Autodesk Fusion 360 part; units mm, degrees
(part 2 of 4)
sketch "Esboço21" plane through (0, 0, 25.51) normal (0, 0, 1) x (-1, 0, 0)
  arc A0 (-264.8266, 72.716) -> (-256.8894, 72.716) centre (-260.858, 77.216) ccw
  line L0 (-264.8266, 72.716) -> (-256.8894, 72.716)
  arc A1 (-203.4723, 131.348) -> (-203.0106, 132.848) centre (-208.9267, 133.848) ccw
  line L1 (-203.4723, 131.348) -> (-214.381, 131.348)
  arc A2 (-214.8427, 132.848) -> (-214.381, 131.348) centre (-208.9267, 133.848) ccw
  line L2 (-214.8427, 132.848) -> (-203.0106, 132.848)
  arc A3 (-212.8953, 129.348) -> (-204.958, 129.348) centre (-208.9267, 133.848) ccw
  line L3 (-212.8953, 129.348) -> (-204.958, 129.348)
  line L4 (-255.4036, 74.716) -> (-266.3124, 74.716)
  arc A4 (-266.7741, 76.216) -> (-266.3124, 74.716) centre (-260.858, 77.216) ccw
  line L5 (-266.7741, 76.216) -> (-254.9419, 76.216)
  arc A5 (-255.4036, 74.716) -> (-254.9419, 76.216) centre (-260.858, 77.216) ccw
  line L6 (-203.0106, 134.848) -> (-214.8427, 134.848)
  arc A6 (-214.381, 136.348) -> (-214.8427, 134.848) centre (-208.9267, 133.848) ccw
  line L7 (-214.381, 136.348) -> (-203.4723, 136.348)
  arc A7 (-203.0106, 134.848) -> (-203.4723, 136.348) centre (-208.9267, 133.848) ccw
  line L8 (-254.9419, 78.216) -> (-266.7741, 78.216)
  arc A8 (-266.3124, 79.716) -> (-266.7741, 78.216) centre (-260.858, 77.216) ccw
  line L9 (-266.3124, 79.716) -> (-255.4036, 79.716)
  arc A9 (-254.9419, 78.216) -> (-255.4036, 79.716) centre (-260.858, 77.216) ccw
  circle A10 centre (-239.522, 60.452) radius 2.5
  circle A11 centre (-207.899, 118.364) radius 2.5
  line L10 (-257.756, 60.626) -> (-257.806, 60.626)
  line L11 (-257.806, 60.626) -> (-257.806, 60.226)
  line L12 (-257.806, 60.226) -> (-265.506, 60.226)
  line L13 (-265.506, 60.226) -> (-265.506, 60.626)
  line L14 (-265.506, 60.626) -> (-265.556, 60.626)
  line L15 (-265.556, 60.626) -> (-265.556, 63.326)
  line L16 (-265.556, 63.326) -> (-265.506, 63.326)
  line L17 (-265.506, 63.326) -> (-265.506, 63.726)
  line L18 (-265.506, 63.726) -> (-257.806, 63.726)
  line L19 (-257.806, 63.726) -> (-257.806, 63.326)
  line L20 (-257.806, 63.326) -> (-257.756, 63.326)
  line L21 (-257.756, 63.326) -> (-257.756, 60.626)
  line L22 (-204.958, 138.348) -> (-212.8953, 138.348)
  arc A12 (-204.958, 138.348) -> (-212.8953, 138.348) centre (-208.9267, 133.848) ccw
  line L23 (-256.8894, 81.716) -> (-264.8266, 81.716)
  arc A13 (-256.8894, 81.716) -> (-264.8266, 81.716) centre (-260.858, 77.216) ccw
  line L24 (-271.5, 38) -> (-166.5, 38)
  line L25 (-166.5, 38) -> (-166.5, 143)
  line L26 (-166.5, 143) -> (-271.5, 143)
  line L27 (-271.5, 143) -> (-271.5, 38)
  spline S0 degree 3 poles (-184.8623, 130.1732) (-186.1405, 129.7688) (-187.3103, 128.5701) (-188.1551, 126.8082) knots 0 0 0 0 1 1 1 1
  spline S1 degree 3 poles (-188.1551, 126.8082) (-188.805, 125.4434) (-189.6138, 123.1543) (-190.1698, 121.118) knots 0 0 0 0 1 1 1 1
  spline S2 degree 3 poles (-190.1698, 121.118) (-190.6175, 119.4716) (-191.5201, 114.6263) (-191.614, 113.3771) knots 0 0 0 0 1 1 1 1
  spline S3 degree 3 poles (-191.614, 113.3771) (-191.7079, 112.1206) (-191.6429, 109.7088) (-191.4985, 109.0589) knots 0 0 0 0 1 1 1 1
  line L28 (-191.4985, 109.0589) -> (-191.3901, 108.6112)
  line L29 (-191.3901, 108.6112) -> (-191.7006, 108.1851)
  spline S4 degree 3 poles (-191.7006, 108.1851) (-191.8667, 107.9541) (-192.0689, 107.6363) (-192.1556, 107.4919) knots 0 0 0 0 1 1 1 1
  line L30 (-192.1556, 107.4919) -> (-192.3072, 107.2175)
  line L31 (-192.3072, 107.2175) -> (-192.6105, 107.788)
  spline S5 degree 3 poles (-192.6105, 107.788) (-193.4842, 109.4127) (-195.0368, 110.8497) (-196.5315, 111.4274) knots 0 0 0 0 1 1 1 1
  spline S6 degree 3 poles (-196.5315, 111.4274) (-197.1742, 111.6729) (-198.1418, 111.8606) (-198.8061, 111.8606) knots 0 0 0 0 1 1 1 1
  spline S7 degree 3 poles (-198.8061, 111.8606) (-199.2611, 111.8606) (-199.2827, 111.8679) (-199.651, 112.2) knots 0 0 0 0 1 1 1 1
  spline S8 degree 3 poles (-199.651, 112.2) (-200.4742, 112.951) (-201.7379, 113.6298) (-202.8355, 113.9186) knots 0 0 0 0 1 1 1 1
  spline S9 degree 3 poles (-202.8355, 113.9186) (-203.0738, 113.9836) (-203.6226, 114.0703) (-204.0631, 114.1136) knots 0 0 0 0 1 1 1 1
  spline S10 degree 3 poles (-204.0631, 114.1136) (-206.5038, 114.3663) (-208.93, 113.3915) (-210.2876, 111.6079) knots 0 0 0 0 1 1 1 1
  spline S11 degree 3 poles (-210.2876, 111.6079) (-211.0386, 110.6258) (-211.5946, 109.2322) (-211.7535, 107.9324) knots 0 0 0 0 1 1 1 1
  spline S12 degree 3 poles (-211.7535, 107.9324) (-211.8762, 106.972) (-211.804, 105.3112) (-211.609, 104.5024) knots 0 0 0 0 1 1 1 1
  spline S13 degree 3 poles (-211.609, 104.5024) (-211.5296, 104.163) (-211.4863, 103.867) (-211.5152, 103.8381) knots 0 0 0 0 1 1 1 1
  spline S14 degree 3 poles (-211.5152, 103.8381) (-211.5513, 103.8164) (-211.8329, 103.737) (-212.1506, 103.6648) knots 0 0 0 0 1 1 1 1
  spline S15 degree 3 poles (-212.1506, 103.6648) (-212.8366, 103.5203) (-214.6491, 102.9282) (-215.5084, 102.5672) knots 0 0 0 0 1 1 1 1
  spline S16 degree 3 poles (-215.5084, 102.5672) (-216.4255, 102.1772) (-216.5627, 102.1989) (-217.8191, 102.8416) knots 0 0 0 0 1 1 1 1
  spline S17 degree 3 poles (-217.8191, 102.8416) (-218.3968, 103.1376) (-219.0467, 103.4265) (-219.2633, 103.477) knots 0 0 0 0 1 1 1 1
  spline S18 degree 3 poles (-219.2633, 103.477) (-219.5089, 103.5348) (-220.2598, 103.5853) (-221.2419, 103.5998) knots 0 0 0 0 1 1 1 1
  line L32 (-221.2419, 103.5998) -> (-222.8161, 103.6214)
  line L33 (-222.8161, 103.6214) -> (-223.3721, 103.9031)
  spline S19 degree 3 poles (-223.3721, 103.9031) (-224.1231, 104.2858) (-224.8163, 104.5024) (-225.459, 104.5602) knots 0 0 0 0 1 1 1 1
  line L34 (-225.459, 104.5602) -> (-226.0006, 104.6035)
  line L35 (-226.0006, 104.6035) -> (-226.4699, 105.6867)
  spline S20 degree 3 poles (-226.4699, 105.6867) (-226.7227, 106.286) (-227.3003, 107.5641) (-227.7481, 108.539) knots 0 0 0 0 1 1 1 1
  spline S21 degree 3 poles (-227.7481, 108.539) (-228.1958, 109.5138) (-228.9756, 111.2035) (-229.4739, 112.2939) knots 0 0 0 0 1 1 1 1
  spline S22 degree 3 poles (-229.4739, 112.2939) (-229.9794, 113.3843) (-230.6148, 114.7346) (-230.8892, 115.2906) knots 0 0 0 0 1 1 1 1
  spline S23 degree 3 poles (-230.8892, 115.2906) (-232.3695, 118.2874) (-234.0304, 120.6414) (-236.1028, 122.6633) knots 0 0 0 0 1 1 1 1
  spline S24 degree 3 poles (-236.1028, 122.6633) (-237.8214, 124.3458) (-239.0345, 125.1546) (-240.9842, 125.92) knots 0 0 0 0 1 1 1 1
  spline S25 degree 3 poles (-240.9842, 125.92) (-242.1901, 126.3894) (-242.7678, 126.5193) (-243.6704, 126.5193) knots 0 0 0 0 1 1 1 1
  spline S26 degree 3 poles (-243.6704, 126.5193) (-246.3061, 126.5193) (-248.2197, 124.909) (-248.2197, 122.685) knots 0 0 0 0 1 1 1 1
  spline S27 degree 3 poles (-248.2197, 122.685) (-248.2197, 121.9268) (-248.1114, 121.4646) (-247.7864, 120.7786) knots 0 0 0 0 1 1 1 1
  spline S28 degree 3 poles (-247.7864, 120.7786) (-247.2737, 119.7316) (-246.8044, 119.3272) (-244.9341, 118.3523) knots 0 0 0 0 1 1 1 1
  spline S29 degree 3 poles (-244.9341, 118.3523) (-243.6777, 117.7025) (-243.4755, 117.5725) (-242.8256, 117.0453) knots 0 0 0 0 1 1 1 1
  spline S30 degree 3 poles (-242.8256, 117.0453) (-241.2875, 115.7961) (-239.6411, 113.7959) (-238.4063, 111.6873) knots 0 0 0 0 1 1 1 1
  spline S31 degree 3 poles (-238.4063, 111.6873) (-237.973, 110.9436) (-237.0704, 109.16) (-236.6516, 108.214) knots 0 0 0 0 1 1 1 1
  spline S32 degree 3 poles (-236.6516, 108.214) (-236.2833, 107.3836) (-235.1496, 104.5674) (-235.1496, 104.488) knots 0 0 0 0 1 1 1 1
  spline S33 degree 3 poles (-235.1496, 104.488) (-235.1496, 104.4519) (-235.4457, 104.423) (-235.7995, 104.423) knots 0 0 0 0 1 1 1 1
  spline S34 degree 3 poles (-235.7995, 104.423) (-236.1606, 104.423) (-236.7021, 104.3724) (-236.9982, 104.3074) knots 0 0 0 0 1 1 1 1
  spline S35 degree 3 poles (-236.9982, 104.3074) (-237.5037, 104.2063) (-237.5614, 104.2063) (-237.7275, 104.3147) knots 0 0 0 0 1 1 1 1
  spline S36 degree 3 poles (-237.7275, 104.3147) (-238.5074, 104.8273) (-240.096, 104.9068) (-241.0781, 104.488) knots 0 0 0 0 1 1 1 1
  line L36 (-241.0781, 104.488) -> (-241.4319, 104.3363)
  line L37 (-241.4319, 104.3363) -> (-242.3129, 104.9068)
  spline S37 degree 3 poles (-242.3129, 104.9068) (-243.5332, 105.6939) (-243.7787, 105.8311) (-244.4359, 106.0549) knots 0 0 0 0 1 1 1 1
  spline S38 degree 3 poles (-244.4359, 106.0549) (-244.9197, 106.2282) (-245.1219, 106.2571) (-245.7645, 106.2571) knots 0 0 0 0 1 1 1 1
  spline S39 degree 3 poles (-245.7645, 106.2571) (-246.6383, 106.2499) (-247.1654, 106.0983) (-247.8803, 105.6217) knots 0 0 0 0 1 1 1 1
  spline S40 degree 3 poles (-247.8803, 105.6217) (-249.5122, 104.5385) (-249.7505, 102.1844) (-248.3858, 100.668) knots 0 0 0 0 1 1 1 1
  spline S41 degree 3 poles (-248.3858, 100.668) (-248.1908, 100.4442) (-247.6276, 100.0181) (-247.0354, 99.621) knots 0 0 0 0 1 1 1 1
  spline S42 degree 3 poles (-247.0354, 99.621) (-246.0534, 98.9783) (-245.2518, 98.4728) (-238.724, 94.3857) knots 0 0 0 0 1 1 1 1
  spline S43 degree 3 poles (-238.724, 94.3857) (-232.7811, 90.6669) (-227.6758, 87.4391) (-227.5459, 87.3091) knots 0 0 0 0 1 1 1 1
  spline S44 degree 3 poles (-227.5459, 87.3091) (-227.5098, 87.2802) (-227.7481, 86.977) (-228.0658, 86.6376) knots 0 0 0 0 1 1 1 1
  spline S45 degree 3 poles (-228.0658, 86.6376) (-228.759, 85.8866) (-229.3583, 85.15) (-229.8783, 84.4207) knots 0 0 0 0 1 1 1 1
  spline S46 degree 3 poles (-229.8783, 84.4207) (-230.0877, 84.1246) (-230.3043, 83.843) (-230.3621, 83.7997) knots 0 0 0 0 1 1 1 1
  spline S47 degree 3 poles (-230.3621, 83.7997) (-230.4776, 83.6986) (-230.687, 83.7491) (-231.4308, 84.0163) knots 0 0 0 0 1 1 1 1
  spline S48 degree 3 poles (-231.4308, 84.0163) (-231.8785, 84.1824) (-232.0518, 84.2041) (-232.8822, 84.2041) knots 0 0 0 0 1 1 1 1
  spline S49 degree 3 poles (-232.8822, 84.2041) (-233.8859, 84.2041) (-234.3336, 84.1102) (-235.0774, 83.7347) knots 0 0 0 0 1 1 1 1
  spline S50 degree 3 poles (-235.0774, 83.7347) (-235.2579, 83.6481) (-235.6767, 83.482) (-236.0161, 83.3737) knots 0 0 0 0 1 1 1 1
  spline S51 degree 3 poles (-236.0161, 83.3737) (-236.3555, 83.2653) (-236.8177, 83.0776) (-237.0487, 82.9548) knots 0 0 0 0 1 1 1 1
  spline S52 degree 3 poles (-237.0487, 82.9548) (-237.807, 82.5577) (-238.5291, 81.6984) (-238.7601, 80.9113) knots 0 0 0 0 1 1 1 1
  spline S53 degree 3 poles (-238.7601, 80.9113) (-238.8396, 80.6513) (-238.8901, 80.6008) (-239.1284, 80.5286) knots 0 0 0 0 1 1 1 1
  spline S54 degree 3 poles (-239.1284, 80.5286) (-239.28, 80.4852) (-239.5833, 80.348) (-239.8072, 80.2325) knots 0 0 0 0 1 1 1 1
  spline S55 degree 3 poles (-239.8072, 80.2325) (-240.5148, 79.8642) (-239.8722, 79.5321) (-245.8728, 83.3231) knots 0 0 0 0 1 1 1 1
  spline S56 degree 3 poles (-245.8728, 83.3231) (-248.5446, 85.0128) (-248.6096, 85.0489) (-248.9851, 85.1861) knots 0 0 0 0 1 1 1 1
  spline S57 degree 3 poles (-248.9851, 85.1861) (-249.5195, 85.3811) (-250.6532, 85.3594) (-251.202, 85.15) knots 0 0 0 0 1 1 1 1
  spline S58 degree 3 poles (-251.202, 85.15) (-252.1985, 84.7601) (-252.9856, 83.9947) (-253.3177, 83.0776) knots 0 0 0 0 1 1 1 1
  spline S59 degree 3 poles (-253.3177, 83.0776) (-253.491, 82.6082) (-253.5055, 82.471) (-253.4766, 81.7995) knots 0 0 0 0 1 1 1 1
  spline S60 degree 3 poles (-253.4766, 81.7995) (-253.4549, 81.1063) (-253.4333, 81.0052) (-253.1805, 80.5069) knots 0 0 0 0 1 1 1 1
  spline S61 degree 3 poles (-253.1805, 80.5069) (-252.5379, 79.1927) (-251.3969, 78.2467) (-248.4002, 76.5137) knots 0 0 0 0 1 1 1 1
  spline S62 degree 3 poles (-248.4002, 76.5137) (-247.7214, 76.1237) (-246.5372, 75.3944) (-245.7645, 74.8889) knots 0 0 0 0 1 1 1 1
  spline S63 degree 3 poles (-245.7645, 74.8889) (-244.9919, 74.3835) (-243.8871, 73.6902) (-243.3094, 73.3364) knots 0 0 0 0 1 1 1 1
  spline S64 degree 3 poles (-243.3094, 73.3364) (-242.7317, 72.9898) (-240.7676, 71.7911) (-238.9407, 70.6791) knots 0 0 0 0 1 1 1 1
  spline S65 degree 3 poles (-238.9407, 70.6791) (-237.1137, 69.567) (-234.998, 68.2817) (-234.247, 67.8195) knots 0 0 0 0 1 1 1 1
  spline S66 degree 3 poles (-234.247, 67.8195) (-233.4888, 67.3646) (-231.9074, 66.3753) (-230.7231, 65.6316) knots 0 0 0 0 1 1 1 1
  spline S67 degree 3 poles (-230.7231, 65.6316) (-228.2752, 64.0791) (-227.8564, 63.8552) (-226.9537, 63.5808) knots 0 0 0 0 1 1 1 1
  spline S68 degree 3 poles (-226.9537, 63.5808) (-226.3761, 63.4075) (-226.1522, 63.3858) (-224.9752, 63.3497) knots 0 0 0 0 1 1 1 1
  spline S69 degree 3 poles (-224.9752, 63.3497) (-223.5671, 63.3136) (-222.9027, 63.3858) (-222.1373, 63.6313) knots 0 0 0 0 1 1 1 1
  line L38 (-222.1373, 63.6313) -> (-221.704, 63.7758)
  line L39 (-221.704, 63.7758) -> (-221.408, 63.5014)
  spline S70 degree 3 poles (-221.408, 63.5014) (-221.2419, 63.3497) (-220.7436, 63.0031) (-220.3104, 62.7359) knots 0 0 0 0 1 1 1 1
  spline S71 degree 3 poles (-220.3104, 62.7359) (-219.8699, 62.4615) (-219.09, 61.9777) (-218.5773, 61.6528) knots 0 0 0 0 1 1 1 1
  spline S72 degree 3 poles (-218.5773, 61.6528) (-218.0574, 61.3278) (-216.8443, 60.5552) (-215.8695, 59.9486) knots 0 0 0 0 1 1 1 1
  spline S73 degree 3 poles (-215.8695, 59.9486) (-214.8946, 59.3348) (-213.3204, 58.3383) (-212.3672, 57.739) knots 0 0 0 0 1 1 1 1
  spline S74 degree 3 poles (-212.3672, 57.739) (-210.3454, 56.4536) (-209.7099, 56.1142) (-208.8073, 55.8543) knots 0 0 0 0 1 1 1 1
  spline S75 degree 3 poles (-208.8073, 55.8543) (-208.1718, 55.6738) (-208.0852, 55.6665) (-206.8215, 55.7027) knots 0 0 0 0 1 1 1 1
  spline S76 degree 3 poles (-206.8215, 55.7027) (-205.4206, 55.7315) (-205.1751, 55.7893) (-204.2436, 56.2587) knots 0 0 0 0 1 1 1 1
  spline S77 degree 3 poles (-204.2436, 56.2587) (-203.2543, 56.7569) (-202.1206, 57.7101) (-201.4346, 58.6127) knots 0 0 0 0 1 1 1 1
  spline S78 degree 3 poles (-201.4346, 58.6127) (-201.2469, 58.8582) (-200.9002, 59.2193) (-200.6692, 59.4215) knots 0 0 0 0 1 1 1 1
  spline S79 degree 3 poles (-200.6692, 59.4215) (-199.3116, 60.5624) (-197.9829, 62.2305) (-197.0442, 63.978) knots 0 0 0 0 1 1 1 1
  spline S80 degree 3 poles (-197.0442, 63.978) (-196.8637, 64.3173) (-196.6976, 64.6134) (-196.6904, 64.6278) knots 0 0 0 0 1 1 1 1
  spline S81 degree 3 poles (-196.6904, 64.6278) (-196.6759, 64.6423) (-196.2355, 64.3751) (-195.7083, 64.0429) knots 0 0 0 0 1 1 1 1
  spline S82 degree 3 poles (-195.7083, 64.0429) (-193.4193, 62.5771) (-192.3578, 61.9344) (-191.7656, 61.6528) knots 0 0 0 0 1 1 1 1
  line L40 (-191.7656, 61.6528) -> (-191.1374, 61.3495)
  line L41 (-191.1374, 61.3495) -> (-190.047, 61.3278)
  spline S83 degree 3 poles (-190.047, 61.3278) (-189.0361, 61.3062) (-188.9133, 61.3134) (-188.3645, 61.4867) knots 0 0 0 0 1 1 1 1
  spline S84 degree 3 poles (-188.3645, 61.4867) (-188.0396, 61.5878) (-187.6496, 61.6744) (-187.498, 61.6744) knots 0 0 0 0 1 1 1 1
  spline S85 degree 3 poles (-187.498, 61.6744) (-186.5737, 61.6744) (-185.245, 62.5626) (-184.6024, 63.6097) knots 0 0 0 0 1 1 1 1
  line L42 (-184.6024, 63.6097) -> (-184.3857, 63.9707)
  line L43 (-184.3857, 63.9707) -> (-182.5227, 64.0068)
  spline S86 degree 3 poles (-182.5227, 64.0068) (-178.3273, 64.1007) (-178.0962, 64.1296) (-177.0853, 64.6351) knots 0 0 0 0 1 1 1 1
  spline S87 degree 3 poles (-177.0853, 64.6351) (-176.5148, 64.9311) (-175.8433, 65.5882) (-175.6122, 66.1009) knots 0 0 0 0 1 1 1 1
  spline S88 degree 3 poles (-175.6122, 66.1009) (-175.3739, 66.6136) (-175.2584, 67.509) (-175.3089, 68.455) knots 0 0 0 0 1 1 1 1
  spline S89 degree 3 poles (-175.3089, 68.455) (-175.3739, 69.8703) (-175.836, 71.0907) (-176.6809, 72.08) knots 0 0 0 0 1 1 1 1
  spline S90 degree 3 poles (-176.6809, 72.08) (-176.9409, 72.376) (-177.1719, 72.701) (-177.208, 72.8021) knots 0 0 0 0 1 1 1 1
  spline S91 degree 3 poles (-177.208, 72.8021) (-177.3525, 73.2425) (-177.2153, 81.2146) (-177.0131, 83.6986) knots 0 0 0 0 1 1 1 1
  spline S92 degree 3 poles (-177.0131, 83.6986) (-176.8542, 85.6916) (-177.1791, 87.0203) (-178.0168, 87.7496) knots 0 0 0 0 1 1 1 1
  spline S93 degree 3 poles (-178.0168, 87.7496) (-178.3562, 88.0529) (-178.9411, 88.3128) (-179.3888, 88.3706) knots 0 0 0 0 1 1 1 1
  line L44 (-179.3888, 88.3706) -> (-179.7426, 88.4067)
  line L45 (-179.7426, 88.4067) -> (-179.7859, 89.1144)
  spline S94 degree 3 poles (-179.7859, 89.1144) (-179.8437, 90.0964) (-180.0892, 90.7969) (-180.5441, 91.2951) knots 0 0 0 0 1 1 1 1
  line L46 (-180.5441, 91.2951) -> (-180.7247, 91.4973)
  line L47 (-180.7247, 91.4973) -> (-180.4647, 92.27)
  spline S95 degree 3 poles (-180.4647, 92.27) (-179.9954, 93.6636) (-179.8365, 94.9562) (-179.9737, 96.1838) knots 0 0 0 0 1 1 1 1
  spline S96 degree 3 poles (-179.9737, 96.1838) (-180.2264, 98.3501) (-181.1652, 99.982) (-182.7538, 101.0219) knots 0 0 0 0 1 1 1 1
  spline S97 degree 3 poles (-182.7538, 101.0219) (-183.4181, 101.4551) (-184.3569, 101.8595) (-184.9634, 101.9678) knots 0 0 0 0 1 1 1 1
  spline S98 degree 3 poles (-184.9634, 101.9678) (-185.7361, 102.1122) (-185.7216, 102.0978) (-185.4617, 102.4733) knots 0 0 0 0 1 1 1 1
  spline S99 degree 3 poles (-185.4617, 102.4733) (-185.1078, 103.0004) (-184.7757, 103.7009) (-184.6096, 104.2785) knots 0 0 0 0 1 1 1 1
  spline S100 degree 3 poles (-184.6096, 104.2785) (-184.4002, 105.0151) (-184.3424, 106.1127) (-184.4796, 106.7698) knots 0 0 0 0 1 1 1 1
  line L48 (-184.4796, 106.7698) -> (-184.5879, 107.2753)
  line L49 (-184.5879, 107.2753) -> (-184.2774, 107.6724)
  spline S101 degree 3 poles (-184.2774, 107.6724) (-183.2448, 109.0228) (-182.7754, 110.3153) (-181.4901, 115.3917) knots 0 0 0 0 1 1 1 1
  spline S102 degree 3 poles (-181.4901, 115.3917) (-181.1724, 116.6482) (-180.7824, 118.1646) (-180.6308, 118.7712) knots 0 0 0 0 1 1 1 1
  spline S103 degree 3 poles (-180.6308, 118.7712) (-179.9304, 121.4935) (-179.656, 123.3565) (-179.7065, 125.1112) knots 0 0 0 0 1 1 1 1
  spline S104 degree 3 poles (-179.7065, 125.1112) (-179.7498, 126.4905) (-179.8726, 127.1115) (-180.2914, 127.9563) knots 0 0 0 0 1 1 1 1
  spline S105 degree 3 poles (-180.2914, 127.9563) (-180.7969, 129.0034) (-181.5912, 129.7038) (-182.7032, 130.0937) knots 0 0 0 0 1 1 1 1
  spline S106 degree 3 poles (-182.7032, 130.0937) (-183.0932, 130.2382) (-183.3315, 130.2671) (-183.8803, 130.2671) knots 0 0 0 0 1 1 1 1
  spline S107 degree 3 poles (-183.8803, 130.2671) (-184.2558, 130.2671) (-184.6962, 130.2237) (-184.8623, 130.1732) knots 0 0 0 0 1 1 1 1
  spline S108 degree 3 poles (-182.9993, 129.1117) (-181.9523, 128.7651) (-181.2301, 127.9347) (-180.8835, 126.6926) knots 0 0 0 0 1 1 1 1
  spline S109 degree 3 poles (-180.8835, 126.6926) (-180.7247, 126.115) (-180.6597, 124.3025) (-180.768, 123.3349) knots 0 0 0 0 1 1 1 1
  spline S110 degree 3 poles (-180.768, 123.3349) (-180.9124, 122.0567) (-181.2013, 120.6125) (-181.6056, 119.0456) knots 0 0 0 0 1 1 1 1
  spline S111 degree 3 poles (-181.6056, 119.0456) (-181.714, 118.6484) (-182.0822, 117.1898) (-182.4361, 115.7961) knots 0 0 0 0 1 1 1 1
  spline S112 degree 3 poles (-182.4361, 115.7961) (-183.1582, 112.951) (-183.7792, 110.7919) (-184.0969, 110.0265) knots 0 0 0 0 1 1 1 1
  spline S113 degree 3 poles (-184.0969, 110.0265) (-184.393, 109.3261) (-184.8768, 108.5173) (-185.3173, 107.9974) knots 0 0 0 0 1 1 1 1
  spline S114 degree 3 poles (-185.3173, 107.9974) (-185.7216, 107.528) (-185.7289, 107.4991) (-185.5844, 107.0153) knots 0 0 0 0 1 1 1 1
  spline S115 degree 3 poles (-185.5844, 107.0153) (-185.1945, 105.73) (-185.5267, 104.0619) (-186.4149, 102.8849) knots 0 0 0 0 1 1 1 1
  spline S116 degree 3 poles (-186.4149, 102.8849) (-187.6352, 101.2602) (-189.5488, 101.0002) (-190.8269, 102.2783) knots 0 0 0 0 1 1 1 1
  spline S117 degree 3 poles (-190.8269, 102.2783) (-191.4768, 102.9282) (-191.9028, 104.1486) (-191.7873, 105.0368) knots 0 0 0 0 1 1 1 1
  spline S118 degree 3 poles (-191.7873, 105.0368) (-191.614, 106.3365) (-191.2602, 107.1958) (-190.6031, 107.9035) knots 0 0 0 0 1 1 1 1
  spline S119 degree 3 poles (-190.6031, 107.9035) (-190.1915, 108.3584) (-190.1915, 108.3584) (-190.4081, 108.9578) knots 0 0 0 0 1 1 1 1
  spline S120 degree 3 poles (-190.4081, 108.9578) (-190.5886, 109.4344) (-190.6897, 110.9508) (-190.6392, 112.3661) knots 0 0 0 0 1 1 1 1
  spline S121 degree 3 poles (-190.6392, 112.3661) (-190.5958, 113.7525) (-190.502, 114.518) (-190.1698, 116.1572) knots 0 0 0 0 1 1 1 1
  spline S122 degree 3 poles (-190.1698, 116.1572) (-190.047, 116.7565) (-189.8665, 117.688) (-189.7726, 118.244) knots 0 0 0 0 1 1 1 1
  spline S123 degree 3 poles (-189.7726, 118.244) (-189.1516, 121.609) (-187.7291, 125.7972) (-186.6459, 127.4364) knots 0 0 0 0 1 1 1 1
  spline S124 degree 3 poles (-186.6459, 127.4364) (-185.6133, 128.9962) (-184.3569, 129.5738) (-182.9993, 129.1117) knots 0 0 0 0 1 1 1 1
  spline S125 degree 3 poles (-242.6595, 125.4073) (-241.9807, 125.2629) (-240.2838, 124.5552) (-239.5617, 124.122) knots 0 0 0 0 1 1 1 1
  spline S126 degree 3 poles (-239.5617, 124.122) (-238.5146, 123.4937) (-237.9008, 123.0027) (-236.6949, 121.7968) knots 0 0 0 0 1 1 1 1
  spline S127 degree 3 poles (-236.6949, 121.7968) (-234.2109, 119.3127) (-232.8317, 117.1753) (-230.687, 112.4744) knots 0 0 0 0 1 1 1 1
  spline S128 degree 3 poles (-230.687, 112.4744) (-230.2465, 111.5212) (-229.6905, 110.3226) (-229.445, 109.8026) knots 0 0 0 0 1 1 1 1
  spline S129 degree 3 poles (-229.445, 109.8026) (-228.9106, 108.6834) (-227.9286, 106.5026) (-227.2137, 104.849) knots 0 0 0 0 1 1 1 1
  line L50 (-227.2137, 104.849) -> (-226.6938, 103.6503)
  line L51 (-226.6938, 103.6503) -> (-226.0583, 103.607)
  spline S130 degree 3 poles (-226.0583, 103.607) (-225.2062, 103.5564) (-224.6358, 103.3904) (-223.7693, 102.9715) knots 0 0 0 0 1 1 1 1
  spline S131 degree 3 poles (-223.7693, 102.9715) (-222.9244, 102.5527) (-222.6572, 102.495) (-222.1518, 102.6177) knots 0 0 0 0 1 1 1 1
  spline S132 degree 3 poles (-222.1518, 102.6177) (-221.8485, 102.6899) (-221.5596, 102.6899) (-220.7509, 102.6249) knots 0 0 0 0 1 1 1 1
  spline S133 degree 3 poles (-220.7509, 102.6249) (-219.5522, 102.5166) (-219.0828, 102.3866) (-218.2524, 101.9245) knots 0 0 0 0 1 1 1 1
  spline S134 degree 3 poles (-218.2524, 101.9245) (-217.2342, 101.3613) (-217.0465, 101.2963) (-216.4471, 101.289) knots 0 0 0 0 1 1 1 1
  spline S135 degree 3 poles (-216.4471, 101.289) (-215.9778, 101.289) (-215.8189, 101.3251) (-215.2629, 101.5562) knots 0 0 0 0 1 1 1 1
  spline S136 degree 3 poles (-215.2629, 101.5562) (-213.8331, 102.1628) (-211.9918, 102.726) (-210.7931, 102.9138) knots 0 0 0 0 1 1 1 1
  spline S137 degree 3 poles (-210.7931, 102.9138) (-210.4753, 102.9571) (-210.2082, 103.0365) (-210.1937, 103.0871) knots 0 0 0 0 1 1 1 1
  spline S138 degree 3 poles (-210.1937, 103.0871) (-210.1721, 103.1304) (-210.2587, 103.4554) (-210.3742, 103.8164) knots 0 0 0 0 1 1 1 1
  spline S139 degree 3 poles (-210.3742, 103.8164) (-210.7931, 105.109) (-210.923, 106.7409) (-210.7064, 108.0696) knots 0 0 0 0 1 1 1 1
  spline S140 degree 3 poles (-210.7064, 108.0696) (-210.3815, 110.0915) (-209.2405, 111.7162) (-207.6014, 112.5105) knots 0 0 0 0 1 1 1 1
  spline S141 degree 3 poles (-207.6014, 112.5105) (-206.6915, 112.951) (-205.9622, 113.1099) (-204.8574, 113.1171) knots 0 0 0 0 1 1 1 1
  spline S142 degree 3 poles (-204.8574, 113.1171) (-202.9727, 113.1243) (-201.5574, 112.5683) (-200.1565, 111.2757) knots 0 0 0 0 1 1 1 1
  spline S143 degree 3 poles (-200.1565, 111.2757) (-199.7449, 110.893) (-199.6799, 110.8786) (-198.5751, 110.8208) knots 0 0 0 0 1 1 1 1
  spline S144 degree 3 poles (-198.5751, 110.8208) (-196.7337, 110.7269) (-195.0584, 109.6943) (-193.8814, 107.9324) knots 0 0 0 0 1 1 1 1
  spline S145 degree 3 poles (-193.8814, 107.9324) (-193.1376, 106.8131) (-192.8416, 105.9899) (-192.6827, 104.6396) knots 0 0 0 0 1 1 1 1
  spline S146 degree 3 poles (-192.6827, 104.6396) (-192.4733, 102.7621) (-192.8705, 100.9858) (-193.7659, 99.8087) knots 0 0 0 0 1 1 1 1
  spline S147 degree 3 poles (-193.7659, 99.8087) (-193.9247, 99.5921) (-194.0619, 99.3755) (-194.0619, 99.3249) knots 0 0 0 0 1 1 1 1
  spline S148 degree 3 poles (-194.0619, 99.3249) (-194.0619, 99.2816) (-193.8092, 99.0794) (-193.4987, 98.8917) knots 0 0 0 0 1 1 1 1
  spline S149 degree 3 poles (-193.4987, 98.8917) (-193.1954, 98.7039) (-192.726, 98.3862) (-192.4589, 98.1912) knots 0 0 0 0 1 1 1 1
  spline S150 degree 3 poles (-192.4589, 98.1912) (-192.1917, 98.0035) (-191.9389, 97.8591) (-191.8956, 97.8879) knots 0 0 0 0 1 1 1 1
  spline S151 degree 3 poles (-191.8956, 97.8879) (-191.8595, 97.9096) (-191.7223, 98.0829) (-191.5996, 98.2706) knots 0 0 0 0 1 1 1 1
  spline S152 degree 3 poles (-191.5996, 98.2706) (-190.7836, 99.4766) (-189.7076, 100.2925) (-188.2923, 100.7763) knots 0 0 0 0 1 1 1 1
  spline S153 degree 3 poles (-188.2923, 100.7763) (-185.9455, 101.5707) (-183.3604, 100.8269) (-182.0389, 98.9711) knots 0 0 0 0 1 1 1 1
  spline S154 degree 3 poles (-182.0389, 98.9711) (-181.2879, 97.9168) (-180.9702, 96.8264) (-180.9702, 95.2884) knots 0 0 0 0 1 1 1 1
  spline S155 degree 3 poles (-180.9702, 95.2884) (-180.9702, 93.938) (-181.2446, 92.7827) (-181.8295, 91.6201) knots 0 0 0 0 1 1 1 1
  line L52 (-181.8295, 91.6201) -> (-182.0245, 91.2446)
  line L53 (-182.0245, 91.2446) -> (-181.8151, 91.1002)
  spline S156 degree 3 poles (-181.8151, 91.1002) (-181.0713, 90.5802) (-180.8619, 90.0748) (-180.7752, 88.645) knots 0 0 0 0 1 1 1 1
  spline S157 degree 3 poles (-180.7752, 88.645) (-180.7463, 88.089) (-180.6958, 87.5763) (-180.6669, 87.5113) knots 0 0 0 0 1 1 1 1
  spline S158 degree 3 poles (-180.6669, 87.5113) (-180.6236, 87.403) (-180.5225, 87.3813) (-180.0531, 87.3813) knots 0 0 0 0 1 1 1 1
  spline S159 degree 3 poles (-180.0531, 87.3813) (-179.3888, 87.3813) (-178.9483, 87.2441) (-178.6306, 86.9336) knots 0 0 0 0 1 1 1 1
  spline S160 degree 3 poles (-178.6306, 86.9336) (-178.1323, 86.4498) (-177.9157, 85.3233) (-178.0312, 83.778) knots 0 0 0 0 1 1 1 1
  spline S161 degree 3 poles (-178.0312, 83.778) (-178.1829, 81.6984) (-178.2551, 79.5682) (-178.2695, 76.297) knots 0 0 0 0 1 1 1 1
  spline S162 degree 3 poles (-178.2695, 76.297) (-178.284, 72.2749) (-178.2984, 72.3832) (-177.6196, 71.6178) knots 0 0 0 0 1 1 1 1
  spline S163 degree 3 poles (-177.6196, 71.6178) (-177.1214, 71.0618) (-176.9264, 70.7585) (-176.7026, 70.1808) knots 0 0 0 0 1 1 1 1
  spline S164 degree 3 poles (-176.7026, 70.1808) (-176.3776, 69.3576) (-176.2693, 68.6716) (-176.3198, 67.7618) knots 0 0 0 0 1 1 1 1
  spline S165 degree 3 poles (-176.3198, 67.7618) (-176.3704, 66.7869) (-176.5293, 66.3609) (-176.9842, 65.9421) knots 0 0 0 0 1 1 1 1
  spline S166 degree 3 poles (-176.9842, 65.9421) (-177.6557, 65.3211) (-178.3345, 65.1261) (-179.9448, 65.09) knots 0 0 0 0 1 1 1 1
  spline S167 degree 3 poles (-179.9448, 65.09) (-180.5803, 65.0828) (-181.5045, 65.0467) (-182.0028, 65.0106) knots 0 0 0 0 1 1 1 1
  spline S168 degree 3 poles (-182.0028, 65.0106) (-182.5011, 64.9817) (-183.3604, 64.9817) (-183.9164, 65.0033) knots 0 0 0 0 1 1 1 1
  spline S169 degree 3 poles (-183.9164, 65.0033) (-184.4724, 65.025) (-184.9634, 65.0322) (-184.9995, 65.0178) knots 0 0 0 0 1 1 1 1
  spline S170 degree 3 poles (-184.9995, 65.0178) (-185.0429, 65.0033) (-185.1728, 64.7723) (-185.2884, 64.5051) knots 0 0 0 0 1 1 1 1
  spline S171 degree 3 poles (-185.2884, 64.5051) (-185.7072, 63.5375) (-186.7615, 62.7432) (-187.7435, 62.6637) knots 0 0 0 0 1 1 1 1
  spline S172 degree 3 poles (-187.7435, 62.6637) (-188.0179, 62.6421) (-188.444, 62.5482) (-188.6823, 62.4688) knots 0 0 0 0 1 1 1 1
  spline S173 degree 3 poles (-188.6823, 62.4688) (-189.2455, 62.2666) (-190.0398, 62.2088) (-190.5958, 62.3243) knots 0 0 0 0 1 1 1 1
  spline S174 degree 3 poles (-190.5958, 62.3243) (-191.2385, 62.4615) (-191.809, 62.772) (-194.423, 64.4257) knots 0 0 0 0 1 1 1 1
  spline S175 degree 3 poles (-194.423, 64.4257) (-195.7155, 65.2416) (-196.842, 65.9493) (-196.9287, 65.9998) knots 0 0 0 0 1 1 1 1
  spline S176 degree 3 poles (-196.9287, 65.9998) (-197.0803, 66.0793) (-197.1092, 66.0504) (-197.4125, 65.4438) knots 0 0 0 0 1 1 1 1
  spline S177 degree 3 poles (-197.4125, 65.4438) (-198.4234, 63.4292) (-199.3622, 62.086) (-200.6403, 60.8296) knots 0 0 0 0 1 1 1 1
  spline S178 degree 3 poles (-200.6403, 60.8296) (-200.9725, 60.5046) (-201.3696, 60.1436) (-201.514, 60.0353) knots 0 0 0 0 1 1 1 1
  spline S179 degree 3 poles (-201.514, 60.0353) (-201.6657, 59.927) (-201.9184, 59.6526) (-202.0773, 59.4359) knots 0 0 0 0 1 1 1 1
  spline S180 degree 3 poles (-202.0773, 59.4359) (-202.8571, 58.3744) (-204.0919, 57.3924) (-205.1679, 56.9591) knots 0 0 0 0 1 1 1 1
  spline S181 degree 3 poles (-205.1679, 56.9591) (-205.6878, 56.7497) (-205.7961, 56.728) (-206.8071, 56.7064) knots 0 0 0 0 1 1 1 1
  spline S182 degree 3 poles (-206.8071, 56.7064) (-208.4173, 56.6703) (-209.0961, 56.8652) (-210.6414, 57.8473) knots 0 0 0 0 1 1 1 1
  spline S183 degree 3 poles (-210.6414, 57.8473) (-211.0314, 58.1) (-212.6055, 59.0893) (-214.1364, 60.0497) knots 0 0 0 0 1 1 1 1
  spline S184 degree 3 poles (-214.1364, 60.0497) (-215.6673, 61.0101) (-217.357, 62.0788) (-217.8913, 62.4182) knots 0 0 0 0 1 1 1 1
  spline S185 degree 3 poles (-217.8913, 62.4182) (-218.4257, 62.7576) (-219.22, 63.2559) (-219.6533, 63.523) knots 0 0 0 0 1 1 1 1
  spline S186 degree 3 poles (-219.6533, 63.523) (-220.592, 64.1007) (-220.8881, 64.3462) (-221.0758, 64.7217) knots 0 0 0 0 1 1 1 1
  spline S187 degree 3 poles (-221.0758, 64.7217) (-221.1552, 64.8734) (-221.2563, 64.9961) (-221.2997, 64.9961) knots 0 0 0 0 1 1 1 1
  spline S188 degree 3 poles (-221.2997, 64.9961) (-221.343, 64.9961) (-221.5885, 64.9095) (-221.8412, 64.8084) knots 0 0 0 0 1 1 1 1
  spline S189 degree 3 poles (-221.8412, 64.8084) (-222.7078, 64.469) (-223.531, 64.3246) (-224.6791, 64.3173) knots 0 0 0 0 1 1 1 1
  spline S190 degree 3 poles (-224.6791, 64.3173) (-225.5456, 64.3173) (-225.8417, 64.3462) (-226.3761, 64.4834) knots 0 0 0 0 1 1 1 1
  spline S191 degree 3 poles (-226.3761, 64.4834) (-227.3003, 64.7217) (-227.7192, 64.9311) (-229.3078, 65.9349) knots 0 0 0 0 1 1 1 1
  spline S192 degree 3 poles (-229.3078, 65.9349) (-231.7341, 67.4802) (-232.5789, 68.0001) (-235.5468, 69.7981) knots 0 0 0 0 1 1 1 1
  spline S193 degree 3 poles (-235.5468, 69.7981) (-240.6304, 72.867) (-243.9448, 74.9106) (-245.4035, 75.8638) knots 0 0 0 0 1 1 1 1
  spline S194 degree 3 poles (-245.4035, 75.8638) (-246.0173, 76.2682) (-247.0715, 76.9181) (-247.7503, 77.308) knots 0 0 0 0 1 1 1 1
  spline S195 degree 3 poles (-247.7503, 77.308) (-250.3643, 78.81) (-251.6569, 79.8209) (-252.1913, 80.7741) knots 0 0 0 0 1 1 1 1
  spline S196 degree 3 poles (-252.1913, 80.7741) (-252.4007, 81.1424) (-252.4368, 81.2868) (-252.4657, 81.7995) knots 0 0 0 0 1 1 1 1
  spline S197 degree 3 poles (-252.4657, 81.7995) (-252.4873, 82.2544) (-252.4657, 82.4855) (-252.379, 82.7165) knots 0 0 0 0 1 1 1 1
  spline S198 degree 3 poles (-252.379, 82.7165) (-251.9602, 83.8069) (-250.7615, 84.5001) (-249.6422, 84.2907) knots 0 0 0 0 1 1 1 1
  spline S199 degree 3 poles (-249.6422, 84.2907) (-249.1512, 84.1969) (-249.1873, 84.2185) (-245.3313, 81.785) knots 0 0 0 0 1 1 1 1
  spline S200 degree 3 poles (-245.3313, 81.785) (-240.4137, 78.68) (-240.9625, 78.9977) (-240.4643, 78.9833) knots 0 0 0 0 1 1 1 1
  spline S201 degree 3 poles (-240.4643, 78.9833) (-240.0888, 78.976) (-239.9588, 79.0122) (-239.5833, 79.2143) knots 0 0 0 0 1 1 1 1
  spline S202 degree 3 poles (-239.5833, 79.2143) (-239.3378, 79.3443) (-238.8973, 79.5248) (-238.6085, 79.6115) knots 0 0 0 0 1 1 1 1
  line L54 (-238.6085, 79.6115) -> (-238.0741, 79.7704)
  line L55 (-238.0741, 79.7704) -> (-237.9225, 80.2397)
  spline S203 degree 3 poles (-237.9225, 80.2397) (-237.5253, 81.4745) (-236.9982, 81.9872) (-235.749, 82.3916) knots 0 0 0 0 1 1 1 1
  spline S204 degree 3 poles (-235.749, 82.3916) (-235.3879, 82.5071) (-234.8319, 82.7165) (-234.5214, 82.861) knots 0 0 0 0 1 1 1 1
  spline S205 degree 3 poles (-234.5214, 82.861) (-233.4166, 83.3592) (-232.6078, 83.3881) (-231.5391, 82.9693) knots 0 0 0 0 1 1 1 1
  spline S206 degree 3 poles (-231.5391, 82.9693) (-231.1058, 82.8032) (-230.8025, 82.731) (-230.5282, 82.731) knots 0 0 0 0 1 1 1 1
  spline S207 degree 3 poles (-230.5282, 82.731) (-229.8566, 82.731) (-229.7844, 82.7743) (-229.3078, 83.4675) knots 0 0 0 0 1 1 1 1
  spline S208 degree 3 poles (-229.3078, 83.4675) (-228.6507, 84.4207) (-227.8925, 85.345) (-226.8815, 86.4137) knots 0 0 0 0 1 1 1 1
  spline S209 degree 3 poles (-226.8815, 86.4137) (-226.3761, 86.9481) (-225.9789, 87.4247) (-226.0006, 87.4752) knots 0 0 0 0 1 1 1 1
  spline S210 degree 3 poles (-226.0006, 87.4752) (-226.0367, 87.5691) (-230.9325, 90.703) (-235.5107, 93.5698) knots 0 0 0 0 1 1 1 1
  spline S211 degree 3 poles (-235.5107, 93.5698) (-248.5952, 101.7584) (-247.5842, 101.0869) (-248.0031, 101.9173) knots 0 0 0 0 1 1 1 1
  spline S212 degree 3 poles (-248.0031, 101.9173) (-248.2991, 102.5094) (-248.3424, 103.0004) (-248.1619, 103.607) knots 0 0 0 0 1 1 1 1
  spline S213 degree 3 poles (-248.1619, 103.607) (-247.9525, 104.2785) (-247.6348, 104.6324) (-246.9416, 104.979) knots 0 0 0 0 1 1 1 1
  spline S214 degree 3 poles (-246.9416, 104.979) (-246.4216, 105.2317) (-246.3567, 105.2534) (-245.7356, 105.2462) knots 0 0 0 0 1 1 1 1
  spline S215 degree 3 poles (-245.7356, 105.2462) (-245.1652, 105.2389) (-245.0063, 105.2101) (-244.5225, 105.0079) knots 0 0 0 0 1 1 1 1
  spline S216 degree 3 poles (-244.5225, 105.0079) (-244.212, 104.8779) (-243.4755, 104.4519) (-242.8761, 104.0619) knots 0 0 0 0 1 1 1 1
  spline S217 degree 3 poles (-242.8761, 104.0619) (-242.2768, 103.6792) (-241.6919, 103.3398) (-241.5763, 103.3109) knots 0 0 0 0 1 1 1 1
  spline S218 degree 3 poles (-241.5763, 103.3109) (-241.4319, 103.2893) (-241.2225, 103.3254) (-240.977, 103.4192) knots 0 0 0 0 1 1 1 1
  spline S219 degree 3 poles (-240.977, 103.4192) (-239.7855, 103.9031) (-239.0201, 103.8814) (-238.0597, 103.3398) knots 0 0 0 0 1 1 1 1
  line L56 (-238.0597, 103.3398) -> (-237.6553, 103.1087)
  line L57 (-237.6553, 103.1087) -> (-236.9765, 103.2676)
  spline S220 degree 3 poles (-236.9765, 103.2676) (-236.11, 103.477) (-235.063, 103.4409) (-234.1531, 103.1737) knots 0 0 0 0 1 1 1 1
  line L58 (-234.1531, 103.1737) -> (-233.5465, 103.0004)
  line L59 (-233.5465, 103.0004) -> (-233.5971, 103.181)
  spline S221 degree 3 poles (-233.5971, 103.181) (-233.6188, 103.282) (-233.9004, 104.0619) (-234.2253, 104.9212) knots 0 0 0 0 1 1 1 1
  spline S222 degree 3 poles (-234.2253, 104.9212) (-236.0306, 109.7593) (-237.7564, 113.016) (-239.8072, 115.4639) knots 0 0 0 0 1 1 1 1
  spline S223 degree 3 poles (-239.8072, 115.4639) (-240.5148, 116.3016) (-242.0385, 117.7747) (-242.6667, 118.2151) knots 0 0 0 0 1 1 1 1
  spline S224 degree 3 poles (-242.6667, 118.2151) (-242.9483, 118.4101) (-243.7426, 118.865) (-244.4286, 119.2333) knots 0 0 0 0 1 1 1 1
  spline S225 degree 3 poles (-244.4286, 119.2333) (-245.8945, 120.006) (-246.2772, 120.2804) (-246.6527, 120.8147) knots 0 0 0 0 1 1 1 1
  spline S226 degree 3 poles (-246.6527, 120.8147) (-247.2521, 121.674) (-247.382, 122.9449) (-246.9632, 123.797) knots 0 0 0 0 1 1 1 1
  spline S227 degree 3 poles (-246.9632, 123.797) (-246.595, 124.5552) (-245.7718, 125.1546) (-244.768, 125.4001) knots 0 0 0 0 1 1 1 1
  spline S228 degree 3 poles (-244.768, 125.4001) (-244.2265, 125.5301) (-243.2444, 125.5301) (-242.6595, 125.4073) knots 0 0 0 0 1 1 1 1
  spline S229 degree 3 poles (-191.419, 101.4262) (-191.2241, 101.2529) (-190.9569, 101.0507) (-190.8269, 100.9785) knots 0 0 0 0 1 1 1 1
  spline S230 degree 3 poles (-190.8269, 100.9785) (-190.7041, 100.9063) (-190.5958, 100.8341) (-190.5958, 100.8125) knots 0 0 0 0 1 1 1 1
  spline S231 degree 3 poles (-190.5958, 100.8125) (-190.5958, 100.7908) (-190.7691, 100.6319) (-190.9785, 100.4586) knots 0 0 0 0 1 1 1 1
  spline S232 degree 3 poles (-190.9785, 100.4586) (-191.1807, 100.2853) (-191.5273, 99.9532) (-191.7368, 99.7149) knots 0 0 0 0 1 1 1 1
  spline S233 degree 3 poles (-191.7368, 99.7149) (-191.9534, 99.4838) (-192.1628, 99.296) (-192.2061, 99.296) knots 0 0 0 0 1 1 1 1
  spline S234 degree 3 poles (-192.2061, 99.296) (-192.2567, 99.296) (-192.3722, 99.361) (-192.4661, 99.4332) knots 0 0 0 0 1 1 1 1
  line L60 (-192.4661, 99.4332) -> (-192.6466, 99.5704)
  line L61 (-192.6466, 99.5704) -> (-192.3144, 100.2853)
  spline S235 degree 3 poles (-192.3144, 100.2853) (-192.1339, 100.6753) (-191.9462, 101.1663) (-191.8956, 101.3757) knots 0 0 0 0 1 1 1 1
  spline S236 degree 3 poles (-191.8956, 101.3757) (-191.8451, 101.5779) (-191.8017, 101.7512) (-191.7873, 101.7512) knots 0 0 0 0 1 1 1 1
  spline S237 degree 3 poles (-191.7873, 101.7512) (-191.7801, 101.7512) (-191.6068, 101.6068) (-191.419, 101.4262) knots 0 0 0 0 1 1 1 1
  spline S238 degree 3 poles (-184.4941, 127.8624) (-185.5628, 127.3642) (-187.3825, 123.2121) (-188.2418, 119.2983) knots 0 0 0 0 1 1 1 1
  spline S239 degree 3 poles (-188.2418, 119.2983) (-189.1949, 114.9873) (-189.4116, 113.3337) (-189.3538, 110.9869) knots 0 0 0 0 1 1 1 1
  spline S240 degree 3 poles (-189.3538, 110.9869) (-189.3105, 109.521) (-189.2311, 109.2322) (-188.7472, 108.6906) knots 0 0 0 0 1 1 1 1
  spline S241 degree 3 poles (-188.7472, 108.6906) (-188.0685, 107.9396) (-187.2886, 107.9252) (-186.4365, 108.6617) knots 0 0 0 0 1 1 1 1
  spline S242 degree 3 poles (-186.4365, 108.6617) (-186.3571, 108.7339) (-186.2054, 108.9072) (-186.1043, 109.0444) knots 0 0 0 0 1 1 1 1
  spline S243 degree 3 poles (-186.1043, 109.0444) (-185.8516, 109.3838) (-184.819, 111.9906) (-184.4146, 113.2976) knots 0 0 0 0 1 1 1 1
  spline S244 degree 3 poles (-184.4146, 113.2976) (-183.9453, 114.7996) (-182.4649, 120.8797) (-182.2483, 122.1939) knots 0 0 0 0 1 1 1 1
  spline S245 degree 3 poles (-182.2483, 122.1939) (-181.7356, 125.2629) (-181.9667, 126.9815) (-182.9921, 127.6964) knots 0 0 0 0 1 1 1 1
  spline S246 degree 3 poles (-182.9921, 127.6964) (-183.2304, 127.8697) (-183.382, 127.913) (-183.7864, 127.9419) knots 0 0 0 0 1 1 1 1
  spline S247 degree 3 poles (-183.7864, 127.9419) (-184.1113, 127.9563) (-184.3496, 127.9347) (-184.4941, 127.8624) knots 0 0 0 0 1 1 1 1
  spline S248 degree 3 poles (-183.4542, 126.3605) (-183.2593, 126.1583) (-183.1943, 125.8261) (-183.1943, 125.039) knots 0 0 0 0 1 1 1 1
  spline S249 degree 3 poles (-183.1943, 125.039) (-183.2015, 123.371) (-183.512, 121.5007) (-184.2702, 118.6845) knots 0 0 0 0 1 1 1 1
  spline S250 degree 3 poles (-184.2702, 118.6845) (-184.3641, 118.3307) (-184.559, 117.5003) (-184.7107, 116.8431) knots 0 0 0 0 1 1 1 1
  spline S251 degree 3 poles (-184.7107, 116.8431) (-184.9562, 115.7456) (-185.7289, 113.0738) (-186.1693, 111.7884) knots 0 0 0 0 1 1 1 1
  spline S252 degree 3 poles (-186.1693, 111.7884) (-186.3426, 111.2757) (-186.9853, 109.9037) (-187.1442, 109.716) knots 0 0 0 0 1 1 1 1
  spline S253 degree 3 poles (-187.1442, 109.716) (-187.1875, 109.6654) (-187.2742, 109.6221) (-187.3464, 109.6221) knots 0 0 0 0 1 1 1 1
  spline S254 degree 3 poles (-187.3464, 109.6221) (-187.4763, 109.6221) (-187.6135, 110.0048) (-187.823, 111.0086) knots 0 0 0 0 1 1 1 1
  spline S255 degree 3 poles (-187.823, 111.0086) (-187.9385, 111.579) (-188.0179, 114.1425) (-187.9024, 113.897) knots 0 0 0 0 1 1 1 1
  spline S256 degree 3 poles (-187.9024, 113.897) (-187.8735, 113.832) (-187.8663, 113.9186) (-187.8879, 114.0992) knots 0 0 0 0 1 1 1 1
  spline S257 degree 3 poles (-187.8879, 114.0992) (-187.9096, 114.3013) (-187.9024, 114.388) (-187.8591, 114.323) knots 0 0 0 0 1 1 1 1
  spline S258 degree 3 poles (-187.8591, 114.323) (-187.7724, 114.193) (-187.6858, 114.8213) (-187.7435, 115.1318) knots 0 0 0 0 1 1 1 1
  spline S259 degree 3 poles (-187.7435, 115.1318) (-187.7796, 115.3051) (-187.7724, 115.334) (-187.7146, 115.2545) knots 0 0 0 0 1 1 1 1
  spline S260 degree 3 poles (-187.7146, 115.2545) (-187.6496, 115.1679) (-187.6352, 115.1895) (-187.6352, 115.3484) knots 0 0 0 0 1 1 1 1
  spline S261 degree 3 poles (-187.6352, 115.3484) (-187.6352, 115.4639) (-187.5847, 115.7311) (-187.5197, 115.9405) knots 0 0 0 0 1 1 1 1
  spline S262 degree 3 poles (-187.5197, 115.9405) (-187.4619, 116.1572) (-187.4186, 116.3738) (-187.4258, 116.4243) knots 0 0 0 0 1 1 1 1
  spline S263 degree 3 poles (-187.4258, 116.4243) (-187.433, 116.4749) (-187.4041, 116.6193) (-187.3536, 116.7348) knots 0 0 0 0 1 1 1 1
  spline S264 degree 3 poles (-187.3536, 116.7348) (-187.303, 116.8576) (-187.2308, 117.1175) (-187.1947, 117.3125) knots 0 0 0 0 1 1 1 1
  spline S265 degree 3 poles (-187.1947, 117.3125) (-187.1586, 117.5147) (-187.0792, 117.8469) (-187.0214, 118.0563) knots 0 0 0 0 1 1 1 1
  spline S266 degree 3 poles (-187.0214, 118.0563) (-186.9564, 118.2657) (-186.9275, 118.4679) (-186.9492, 118.5112) knots 0 0 0 0 1 1 1 1
  spline S267 degree 3 poles (-186.9492, 118.5112) (-186.9781, 118.5473) (-186.9636, 118.6195) (-186.9275, 118.6701) knots 0 0 0 0 1 1 1 1
  spline S268 degree 3 poles (-186.9275, 118.6701) (-186.8842, 118.7206) (-186.7542, 119.1467) (-186.6243, 119.616) knots 0 0 0 0 1 1 1 1
  spline S269 degree 3 poles (-186.6243, 119.616) (-186.4437, 120.302) (-186.4149, 120.4898) (-186.4943, 120.5331) knots 0 0 0 0 1 1 1 1
  spline S270 degree 3 poles (-186.4943, 120.5331) (-186.5665, 120.5764) (-186.5521, 120.5981) (-186.451, 120.5981) knots 0 0 0 0 1 1 1 1
  spline S271 degree 3 poles (-186.451, 120.5981) (-186.3715, 120.5981) (-186.3282, 120.6198) (-186.3499, 120.6414) knots 0 0 0 0 1 1 1 1
  spline S272 degree 3 poles (-186.3499, 120.6414) (-186.3787, 120.6631) (-186.3354, 120.8147) (-186.2632, 120.9808) knots 0 0 0 0 1 1 1 1
  spline S273 degree 3 poles (-186.2632, 120.9808) (-186.0971, 121.3707) (-186.0033, 121.7896) (-186.1043, 121.7246) knots 0 0 0 0 1 1 1 1
  spline S274 degree 3 poles (-186.1043, 121.7246) (-186.1477, 121.6957) (-186.1621, 121.739) (-186.1405, 121.8329) knots 0 0 0 0 1 1 1 1
  spline S275 degree 3 poles (-186.1405, 121.8329) (-186.1116, 121.934) (-186.0827, 121.9556) (-186.0466, 121.8979) knots 0 0 0 0 1 1 1 1
  spline S276 degree 3 poles (-186.0466, 121.8979) (-186.0177, 121.8473) (-185.9094, 122.064) (-185.8011, 122.3961) knots 0 0 0 0 1 1 1 1
  spline S277 degree 3 poles (-185.8011, 122.3961) (-185.6927, 122.7211) (-185.6278, 123.0171) (-185.6494, 123.0532) knots 0 0 0 0 1 1 1 1
  spline S278 degree 3 poles (-185.6494, 123.0532) (-185.6711, 123.0966) (-185.6566, 123.1254) (-185.6133, 123.1254) knots 0 0 0 0 1 1 1 1
  spline S279 degree 3 poles (-185.6133, 123.1254) (-185.5628, 123.1254) (-185.5411, 123.176) (-185.57, 123.2338) knots 0 0 0 0 1 1 1 1
  spline S280 degree 3 poles (-185.57, 123.2338) (-185.5917, 123.2915) (-185.5844, 123.3421) (-185.5483, 123.3421) knots 0 0 0 0 1 1 1 1
  spline S281 degree 3 poles (-185.5483, 123.3421) (-185.4617, 123.3421) (-185.3028, 123.7537) (-185.3606, 123.8403) knots 0 0 0 0 1 1 1 1
  spline S282 degree 3 poles (-185.3606, 123.8403) (-185.3822, 123.8837) (-185.375, 123.9198) (-185.3389, 123.9198) knots 0 0 0 0 1 1 1 1
  spline S283 degree 3 poles (-185.3389, 123.9198) (-185.2306, 123.9198) (-185.0284, 124.4758) (-185.0862, 124.613) knots 0 0 0 0 1 1 1 1
  spline S284 degree 3 poles (-185.0862, 124.613) (-185.1151, 124.6924) (-185.1006, 124.7213) (-185.0573, 124.6924) knots 0 0 0 0 1 1 1 1
  spline S285 degree 3 poles (-185.0573, 124.6924) (-184.9634, 124.6346) (-184.8695, 124.8368) (-184.9418, 124.9452) knots 0 0 0 0 1 1 1 1
  spline S286 degree 3 poles (-184.9418, 124.9452) (-184.9634, 124.9957) (-184.949, 125.0029) (-184.9057, 124.974) knots 0 0 0 0 1 1 1 1
  spline S287 degree 3 poles (-184.9057, 124.974) (-184.8551, 124.9452) (-184.8118, 124.974) (-184.8046, 125.0535) knots 0 0 0 0 1 1 1 1
  spline S288 degree 3 poles (-184.8046, 125.0535) (-184.8046, 125.1257) (-184.7901, 125.2195) (-184.7901, 125.2557) knots 0 0 0 0 1 1 1 1
  spline S289 degree 3 poles (-184.7901, 125.2557) (-184.7829, 125.299) (-184.7251, 125.4073) (-184.6529, 125.5084) knots 0 0 0 0 1 1 1 1
  spline S290 degree 3 poles (-184.6529, 125.5084) (-184.5879, 125.6023) (-184.5302, 125.7395) (-184.5302, 125.8045) knots 0 0 0 0 1 1 1 1
  spline S291 degree 3 poles (-184.5302, 125.8045) (-184.5302, 125.8622) (-184.4074, 126.05) (-184.2558, 126.2161) knots 0 0 0 0 1 1 1 1
  spline S292 degree 3 poles (-184.2558, 126.2161) (-183.9308, 126.5627) (-183.6781, 126.606) (-183.4542, 126.3605) knots 0 0 0 0 1 1 1 1
  spline S293 degree 3 poles (-185.9527, 122.1506) (-185.9744, 122.0856) (-186.0105, 122.0495) (-186.0249, 122.0712) knots 0 0 0 0 1 1 1 1
  spline S294 degree 3 poles (-186.0249, 122.0712) (-186.0466, 122.0928) (-186.0394, 122.1362) (-186.0105, 122.1795) knots 0 0 0 0 1 1 1 1
  spline S295 degree 3 poles (-186.0105, 122.1795) (-185.9455, 122.295) (-185.9022, 122.2734) (-185.9527, 122.1506) knots 0 0 0 0 1 1 1 1
  spline S296 degree 3 poles (-186.6459, 120.006) (-186.6676, 119.9482) (-186.6893, 119.9699) (-186.6893, 120.0493) knots 0 0 0 0 1 1 1 1
  spline S297 degree 3 poles (-186.6893, 120.0493) (-186.6965, 120.1287) (-186.6748, 120.172) (-186.6531, 120.1432) knots 0 0 0 0 1 1 1 1
  spline S298 degree 3 poles (-186.6531, 120.1432) (-186.6315, 120.1215) (-186.6243, 120.0565) (-186.6459, 120.006) knots 0 0 0 0 1 1 1 1
  spline S299 degree 3 poles (-187.0142, 118.309) (-187.0864, 118.2368) (-187.1514, 118.3451) (-187.0864, 118.439) knots 0 0 0 0 1 1 1 1
  spline S300 degree 3 poles (-187.0864, 118.439) (-187.0431, 118.5184) (-187.0286, 118.5184) (-186.9998, 118.439) knots 0 0 0 0 1 1 1 1
  spline S301 degree 3 poles (-186.9998, 118.439) (-186.9853, 118.3885) (-186.9925, 118.3307) (-187.0142, 118.309) knots 0 0 0 0 1 1 1 1
  spline S302 degree 3 poles (-187.5124, 116.251) (-187.5341, 116.1933) (-187.5558, 116.2149) (-187.5558, 116.2944) knots 0 0 0 0 1 1 1 1
  spline S303 degree 3 poles (-187.5558, 116.2944) (-187.563, 116.3738) (-187.5413, 116.4171) (-187.5197, 116.3882) knots 0 0 0 0 1 1 1 1
  spline S304 degree 3 poles (-187.5197, 116.3882) (-187.498, 116.3666) (-187.4908, 116.3016) (-187.5124, 116.251) knots 0 0 0 0 1 1 1 1
  spline S305 degree 3 poles (-188.7761, 107.7085) (-189.8376, 107.2175) (-190.5958, 105.8744) (-190.502, 104.654) knots 0 0 0 0 1 1 1 1
  spline S306 degree 3 poles (-190.502, 104.654) (-190.4009, 103.3182) (-189.5632, 102.5455) (-188.5234, 102.8271) knots 0 0 0 0 1 1 1 1
  spline S307 degree 3 poles (-188.5234, 102.8271) (-187.8735, 103.0004) (-187.1153, 103.968) (-186.812, 104.9934) knots 0 0 0 0 1 1 1 1
  spline S308 degree 3 poles (-186.812, 104.9934) (-186.682, 105.4411) (-186.6604, 106.2066) (-186.7687, 106.6037) knots 0 0 0 0 1 1 1 1
  spline S309 degree 3 poles (-186.7687, 106.6037) (-186.8914, 107.0442) (-187.2814, 107.5497) (-187.6352, 107.7302) knots 0 0 0 0 1 1 1 1
  spline S310 degree 3 poles (-187.6352, 107.7302) (-188.0468, 107.9324) (-188.2995, 107.9324) (-188.7761, 107.7085) knots 0 0 0 0 1 1 1 1
  spline S311 degree 3 poles (-188.0396, 106.3582) (-187.6208, 105.6867) (-188.1479, 104.0042) (-188.6967, 104.2424) knots 0 0 0 0 1 1 1 1
  spline S312 degree 3 poles (-188.6967, 104.2424) (-188.7689, 104.2785) (-188.8556, 104.293) (-188.8989, 104.2858) knots 0 0 0 0 1 1 1 1
  spline S313 degree 3 poles (-188.8989, 104.2858) (-188.935, 104.2713) (-188.9494, 104.293) (-188.9205, 104.3219) knots 0 0 0 0 1 1 1 1
  spline S314 degree 3 poles (-188.9205, 104.3219) (-188.8917, 104.3508) (-188.9061, 104.423) (-188.9567, 104.4807) knots 0 0 0 0 1 1 1 1
  spline S315 degree 3 poles (-188.9567, 104.4807) (-189.065, 104.6179) (-189.0794, 105.8383) (-188.9711, 106.0477) knots 0 0 0 0 1 1 1 1
  spline S316 degree 3 poles (-188.9711, 106.0477) (-188.805, 106.3654) (-188.6245, 106.5171) (-188.379, 106.5171) knots 0 0 0 0 1 1 1 1
  spline S317 degree 3 poles (-188.379, 106.5171) (-188.2129, 106.5171) (-188.1118, 106.4665) (-188.0396, 106.3582) knots 0 0 0 0 1 1 1 1
  spline S318 degree 3 poles (-189.1011, 105.5639) (-189.1227, 105.5133) (-189.1372, 105.5495) (-189.1372, 105.6505) knots 0 0 0 0 1 1 1 1
  spline S319 degree 3 poles (-189.1372, 105.6505) (-189.1372, 105.7516) (-189.1227, 105.7877) (-189.1011, 105.7444) knots 0 0 0 0 1 1 1 1
  spline S320 degree 3 poles (-189.1011, 105.7444) (-189.0866, 105.6939) (-189.0866, 105.6072) (-189.1011, 105.5639) knots 0 0 0 0 1 1 1 1
  spline S321 degree 3 poles (-189.1733, 105.0223) (-189.1949, 104.9501) (-189.2094, 104.9934) (-189.2094, 105.109) knots 0 0 0 0 1 1 1 1
  spline S322 degree 3 poles (-189.2094, 105.109) (-189.2094, 105.2317) (-189.1949, 105.2823) (-189.1733, 105.2389) knots 0 0 0 0 1 1 1 1
  spline S323 degree 3 poles (-189.1733, 105.2389) (-189.1588, 105.1884) (-189.1588, 105.0873) (-189.1733, 105.0223) knots 0 0 0 0 1 1 1 1
  spline S324 degree 3 poles (-244.8258, 124.1725) (-245.2085, 124.0497) (-245.714, 123.6454) (-245.8873, 123.3132) knots 0 0 0 0 1 1 1 1
  spline S325 degree 3 poles (-245.8873, 123.3132) (-245.9595, 123.176) (-246.01, 122.916) (-246.01, 122.6489) knots 0 0 0 0 1 1 1 1
  spline S326 degree 3 poles (-246.01, 122.6489) (-246.01, 121.7823) (-245.7284, 121.5152) (-243.4755, 120.2731) knots 0 0 0 0 1 1 1 1
  spline S327 degree 3 poles (-243.4755, 120.2731) (-242.9122, 119.9626) (-242.1612, 119.4933) (-241.8146, 119.2333) knots 0 0 0 0 1 1 1 1
  spline S328 degree 3 poles (-241.8146, 119.2333) (-240.9192, 118.5618) (-239.5183, 117.1753) (-238.6879, 116.1427) knots 0 0 0 0 1 1 1 1
  spline S329 degree 3 poles (-238.6879, 116.1427) (-237.1282, 114.2075) (-235.5107, 111.4707) (-234.608, 109.225) knots 0 0 0 0 1 1 1 1
  spline S330 degree 3 poles (-234.608, 109.225) (-233.2144, 105.7877) (-232.6656, 104.3941) (-232.2973, 103.412) knots 0 0 0 0 1 1 1 1
  spline S331 degree 3 poles (-232.2973, 103.412) (-232.0662, 102.7982) (-231.7991, 102.2061) (-231.7124, 102.0978) knots 0 0 0 0 1 1 1 1
  spline S332 degree 3 poles (-231.7124, 102.0978) (-231.6257, 101.9895) (-231.3658, 101.549) (-231.1347, 101.123) knots 0 0 0 0 1 1 1 1